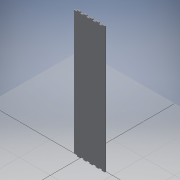
# Autodesk Inventor part: низ
Saved by Autodesk Inventor 2019 (Build 230136000, 136)
## iProperties
Created: 2022-06-29
Part Number: низ
Material: Типовые
Document SubType Name: Modeling
Designer: korsh
Density: 1 g/cm^3
Appearance: По умолчанию
Author: korsh
Autodesk Inventor part; units mm, degrees
ref_plane "YZ Plane" through (0, 0, 0) normal (1, 0, 0) x (0, 1, 0)
ref_plane "XZ Plane" through (0, 0, 0) normal (0, 1, 0) x (-1, 0, 0)
ref_plane "XY Plane" through (0, 0, 0) normal (0, 0, 1) x (1, 0, 0)
sketch "Эскиз1" plane through (0, 0, 0) normal (0, 0, 1) x (1, 0, 0)
  line L0 (0, 0) -> (-10, 0) projected
  line L1 (0, 0) -> (0, 4) projected
  line L2 (-10, 4) -> (0, 4) projected
  line L3 (-10, 0) -> (-10, 4) projected
  line L4 (20, 0) -> (10, 0) projected
  line L5 (20, 0) -> (20, 4) projected
  line L6 (10, 4) -> (20, 4) projected
  line L7 (10, 0) -> (10, 4) projected
  line L8 (-20, 4) -> (-10, 4) projected
  line L9 (0, 4) -> (10, 4) projected
  line L10 (40, 0) -> (30, 0) projected
  line L11 (40, 0) -> (40, 4) projected
  line L12 (30, 4) -> (40, 4) projected
  line L13 (30, 0) -> (30, 4) projected
  line L14 (20, 4) -> (30, 4) projected
  line L15 (40, 4) -> (50, 4) projected
  line L16 (60, 0) -> (50, 0) projected
  line L17 (60, 0) -> (60, 4) projected
  line L18 (50, 4) -> (60, 4) projected
  line L19 (50, 0) -> (50, 4) projected
  line L20 (60, 4) -> (70, 4) projected
  line L21 (80, 0) -> (70, 0) projected
  line L22 (80, 4) -> (80, 0) projected
  line L23 (70, 4) -> (80, 4) projected
  line L24 (70, 0) -> (70, 4) projected
  line L25 (-20, 404) -> (-10, 404) projected
  line L26 (0, 404) -> (10, 404) projected
  line L27 (20, 404) -> (30, 404) projected
  line L28 (40, 404) -> (50, 404) projected
  line L29 (60, 404) -> (70, 404) projected
  line L30 (80, 404) -> (70, 404) projected
  line L31 (80, 408) -> (80, 404) projected
  line L32 (70, 408) -> (80, 408) projected
  line L33 (70, 404) -> (70, 408) projected
  line L34 (60, 404) -> (50, 404) projected
  line L35 (60, 404) -> (60, 408) projected
  line L36 (50, 408) -> (60, 408) projected
  line L37 (50, 404) -> (50, 408) projected
  line L38 (40, 404) -> (30, 404) projected
  line L39 (40, 404) -> (40, 408) projected
  line L40 (30, 408) -> (40, 408) projected
  line L41 (30, 404) -> (30, 408) projected
  line L42 (10, 408) -> (20, 408) projected
  line L43 (20, 404) -> (10, 404) projected
  line L44 (20, 404) -> (20, 408) projected
  line L45 (10, 408) -> (20, 408) projected
  line L46 (10, 404) -> (10, 408) projected
  line L47 (0, 404) -> (-10, 404) projected
  line L48 (0, 404) -> (0, 408) projected
  line L49 (-10, 408) -> (0, 408) projected
  line L50 (-10, 404) -> (-10, 408) projected
  line L51 (80, 4) -> (80, 404)
  line L52 (-20, 4) -> (-20, 404)
  constraints: 4 end point, 1 collinear, 1 parallel
extrude "Выдавливание1" add sketch "Эскиз1" along normal blind 4
